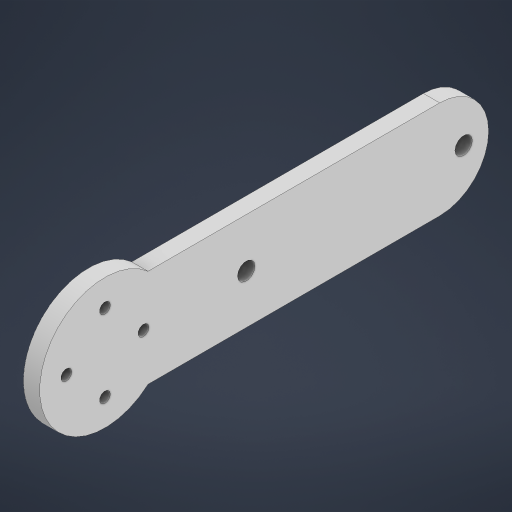
# Autodesk Inventor part: union_servos_2
Saved by Autodesk Inventor 2023.1 (Build 271208000, 208)
## iProperties
Created: 2022-11-07
Part Number: union_servos_2
Material: Generic
Document SubType Name: Modeling
Designer: amtat
Density: 1 g/cm^3
Appearance: Default
Author: amtat
Autodesk Inventor part; units mm, degrees
ref_plane "YZ Plane" through (0, 0, 0) normal (1, 0, 0) x (0, 1, 0)
ref_plane "XZ Plane" through (0, 0, 0) normal (0, 1, 0) x (-1, 0, 0)
ref_plane "XY Plane" through (0, 0, 0) normal (0, 0, 1) x (1, 0, 0)
sketch "Sketch1" plane through (0, 0, 0) normal (1, 0, 0) x (0, 1, 0)
  circle A0 centre (0, 0) radius 1.6
  line L0 (0, 0) -> (0, -40)
  circle A1 centre (0, -40) radius 1.6
  line L1 (0, -40) -> (0, -44.6)
  line L2 (0, -44.6) -> (0, -35.6)
  line L3 (0, 0) -> (0, 4.6)
  line L4 (0, 4.6) -> (0, -4.4)
  circle A2 centre (0, -35.6) radius 9
  line L5 (9, -4.4) -> (9, -35.6)
  line L6 (-9, -35.6) -> (-9, -4.4)
  line L7 (0, 0) -> (0, 7)
  line L8 (0, 7) -> (9, 7)
  line L9 (9, 7) -> (9, -4.4)
  line L10 (0, 7) -> (-9, 7)
  line L11 (-9, 7) -> (-9, -4.4)
  dimension "d0" = 3.2
  dimension "d1" = 40
  dimension "d2" = 3.2
  dimension "d3" = 4.6
  dimension "d4" = 9
  dimension "d5" = 4.6
  dimension "d6" = 9
  dimension "d9" = 7
  constraints: 24 end point, 4 point on line, 3 centre point, 3 coincident, 3 perpendicular, 3 point on circle, 3 vertical, 1 tangent
  measures "d0" diameter of A0
  measures "d1" distance of L0.start L0.end
  measures "d2" diameter of A1
  measures "d3" distance of L1.start L1.end
  measures "d4" distance of L1.end L2.end
  measures "d5" distance of L0.start L3.end
  measures "d6" distance of L3.end L4.end
  measures "d9" distance of L0.start L7.end
extrude "Extrusion2" add sketch "Sketch1" along normal blind 3 contours A0 L3 L7 L8 L9 L5 A2 L0 | A0 L0 A2 L6 L11 L10 L7 L3 | A2 L1 A1 L0 | L0 A1 L1 A2
sketch "Sketch2" plane through (0, -9, 7) normal (0, 0, 1) x (1, 0, 0)
  line L0 (0, 18) -> (0, 0) projected
  line L1 (0, 0) -> (3, 0) projected
  line L2 (3, 18) -> (3, 0) projected
  line L3 (0, 18) -> (3, 18) projected
  point P0 (0, 9)
extrude "Extrusion3" add sketch "Sketch2" along normal blind 24.5
sketch "Sketch5" plane through (3, 0, 0) normal (1, 0, 0) x (0, 0, -1)
  line L0 (35.6, 9) -> (-31.5, 9) projected
  line L1 (-31.5, -9) -> (-31.5, 9) projected
  line L2 (35.6, -9) -> (-31.5, -9) projected
  arc A0 (35.6, -9) -> (35.6, 9) centre (35.6, 0) ccw projected
  circle A1 centre (40, 0) radius 1.6 projected
  circle A2 centre (0, 0) radius 1.6 projected
  line L3 (0, 0) -> (-10, 0)
  line L4 (-10, 0) -> (-10, 9)
  line L5 (35.6, 9) -> (-31.5, 9) projected
  line L6 (-10, 0) -> (-10, -9)
  line L7 (35.6, -9) -> (-31.5, -9) projected
  line L8 (-10, -9) -> (-14, -9)
  line L9 (-14, -9) -> (-14, 9)
  line L10 (-10, 9) -> (-14, 9)
  dimension "d18" = 10
  dimension "d19" = 4
  constraints: 12 end point, 5 point on line, 2 perpendicular, 1 collinear, 1 horizontal
  measures "d18" distance of L3.start L3.end
  measures "d19" distance of L6.end L8.end
extrude "Extrusion5" add sketch "Sketch5" along normal blind 4.3 contours L4 L6 L2 L9 L0
sketch "Sketch6" plane through (7.3, 0, 0) normal (1, 0, 0) x (0, 0, -1)
  line L0 (-14, -9) -> (-10, -9) projected
  line L1 (-10, -9) -> (-10, 9) projected
  line L2 (-10, 9) -> (-14, 9) projected
  line L3 (-14, 9) -> (-14, -9) projected
  line L4 (-14, -9) -> (-14, 9) projected
  line L5 (-14, 9) -> (-14, 0)
  line L6 (-14, 0) -> (-26, 0)
  circle A0 centre (-26, 0) radius 12
  line L7 (-14, 9) -> (-18.0627, 9)
  line L8 (-14, 9) -> (-31.5, 9) projected
  line L9 (-14, -9) -> (-18.0627, -9)
  line L10 (-14, -9) -> (-31.5, -9) projected
  point P0 (0, 0)
  dimension "d22" = 12
  constraints: 8 end point, 3 point on circle, 2 point on line, 1 centre point, 1 coincident, 1 midpoint, 1 perpendicular
  measures "d22" distance of L5.end L6.end
extrude "Extrusion6" add sketch "Sketch6" along normal blind 3
sketch "Sketch7" plane through (0, 0, 0) normal (-1, 0, 0) x (0, 0, 1)
  line L0 (10, -9) -> (10, 9) projected
  line L1 (14, 9) -> (14, -9) projected
  line L2 (-35.6, 9) -> (31.5, 9) projected
  line L3 (-35.6, 9) -> (31.5, 9) projected
  arc A0 (-35.6, 9) -> (-35.6, -9) centre (-35.6, 0) ccw projected
  line L4 (-35.6, -9) -> (31.5, -9) projected
  line L5 (31.5, 9) -> (31.5, -9) projected
  circle A1 centre (-40, 0) radius 1.6 projected
  circle A2 centre (0, 0) radius 1.6 projected
extrude "Extrusion7" add sketch "Sketch7" along normal blind 2.7 contours L0 L2 L1 L4
sketch "Sketch8" plane through (-2.7, 0, 0) normal (-1, 0, 0) x (0, 0, 1)
  line L0 (14, -9) -> (14, 9) projected
  line L1 (14, 9) -> (10, 9) projected
  line L2 (10, 9) -> (10, -9) projected
  line L3 (10, -9) -> (14, -9) projected
  line L4 (14, 9) -> (14, -9) projected
  line L5 (18.0627, -9) -> (14, -9) projected
  arc A0 (18.0627, -9) -> (18.0627, 9) centre (26, 0) ccw projected
  line L6 (14, 9) -> (18.0627, 9) projected
  point P0 (0, 0)
extrude "Extrusion8" add sketch "Sketch8" along normal blind 3
sketch "Sketch9" plane through (0, -9, 31.5) normal (0, 0, 1) x (1, 0, 0)
  line L0 (0, 18) -> (0, 0) projected
  line L1 (0, 0) -> (3, 0) projected
  line L2 (3, 0) -> (3, 18) projected
  line L3 (3, 18) -> (0, 18) projected
  point P0 (0, 9)
extrude "Extrusion9" cut sketch "Sketch9" against normal blind 17.5
sketch "Sketch10" plane through (10.3, 0, 0) normal (1, 0, 0) x (0, 0, -1)
  line L0 (-18.0627, -9) -> (-10, -9) projected
  line L1 (-10, -9) -> (-10, 9) projected
  line L2 (-10, 9) -> (-18.0627, 9) projected
  arc A0 (-18.0627, 9) -> (-18.0627, -9) centre (-26, 0) ccw projected
  circle A1 centre (-26, 0) radius 12
  line L3 (-26, 0) -> (-18.9, 0)
  line L4 (-26, 0) -> (-26, -7.1)
  circle A2 centre (-18.9, 0) radius 1
  circle A3 centre (-26, -7.1) radius 1
  circle A4 centre (-33.1, 0) radius 1
  circle A5 centre (-26, 7.1) radius 1
  point P0 (0, 0)
  dimension "d31" = 7.1
  dimension "d32" = 7.1
  dimension "d33" = 2
  dimension "d34" = 2
  constraints: 5 centre point, 4 end point, 3 coincident, 2 symmetric about line, 1 concentric, 1 horizontal, 1 vertical, 2 other
  measures "d31" distance of L3.start L3.end
  measures "d32" distance of L3.start L4.end
  measures "d33" diameter of A2
  measures "d34" diameter of A3
extrude "Extrusion10" cut sketch "Sketch10" against normal blind 17.5 contours A2 | A3 | A4 | A5
sketch "Sketch11" plane through (-5.7, 0, 0) normal (-1, 0, 0) x (0, 0, 1)
  circle A0 centre (26, -7.1) radius 1 projected
  circle A1 centre (26, 7.1) radius 1 projected
  circle A2 centre (33.1, 0) radius 1 projected
  circle A3 centre (18.9, 0) radius 1 projected
  line L0 (18.0627, 9) -> (10, 9) projected
  line L1 (10, 9) -> (10, -9) projected
  line L2 (10, -9) -> (18.0627, -9) projected
  arc A4 (18.0627, -9) -> (18.0627, 9) centre (26, 0) ccw projected
  point P0 (0, 0)
extrude "Extrusion11" add sketch "Sketch11" along normal blind 1.7
sketch "Sketch12" plane through (-2.7, 0, 0) normal (1, 0, 0) x (0, 0, -1)
  circle A0 centre (-26, -7.1) radius 1 projected
  circle A1 centre (-26, 7.1) radius 1 projected
  circle A2 centre (-33.1, 0) radius 1 projected
  circle A3 centre (-18.9, 0) radius 1 projected
  line L0 (-18.0627, -9) -> (-10, -9) projected
  line L1 (-10, -9) -> (-10, 9) projected
  line L2 (-10, 9) -> (-18.0627, 9) projected
  arc A4 (-18.0627, 9) -> (-18.0627, -9) centre (-26, 0) ccw projected
  circle A5 centre (-26, -7.1) radius 1 projected
  circle A6 centre (-26, 7.1) radius 1 projected
  circle A7 centre (-33.1, 0) radius 1 projected
  circle A8 centre (-18.9, 0) radius 1 projected
  line L3 (-14, -9) -> (-14, 9) projected
  line L4 (-18.0627, 9) -> (-14, 9) projected
  arc A9 (-18.0627, 9) -> (-18.0627, -9) centre (-26, 0) ccw projected
  line L5 (-14, -9) -> (-18.0627, -9) projected
  point P0 (0, 0)
extrude "Extrusion12" cut sketch "Sketch12" against normal blind 1.7 contours A4 L2 L3 L0
sketch "Sketch13" plane through (10.3, 0, 0) normal (1, 0, 0) x (0, 0, -1)
  circle A0 centre (-26, -7.1) radius 1 projected
  circle A1 centre (-26, 7.1) radius 1 projected
  circle A2 centre (-33.1, 0) radius 1 projected
  circle A3 centre (-18.9, 0) radius 1 projected
  line L0 (-18.0627, -9) -> (-10, -9) projected
  line L1 (-10, -9) -> (-10, 9) projected
  line L2 (-10, 9) -> (-18.0627, 9) projected
  arc A4 (-18.0627, 9) -> (-18.0627, -9) centre (-26, 0) ccw projected
  point P0 (0, 0)
extrude "Extrusion13" add sketch "Sketch13" along normal blind 1.7
sketch "Sketch14" plane through (7.3, 0, 0) normal (-1, 0, 0) x (0, 0, 1)
  line L0 (10, -9) -> (10, 9) projected
  line L1 (10, 9) -> (18.0627, 9) projected
  arc A0 (18.0627, -9) -> (18.0627, 9) centre (26, 0) ccw projected
  line L2 (18.0627, -9) -> (10, -9) projected
  circle A1 centre (18.9, 0) radius 1 projected
  circle A2 centre (33.1, 0) radius 1 projected
  circle A3 centre (26, 7.1) radius 1 projected
  circle A4 centre (26, -7.1) radius 1 projected
  circle A5 centre (26, -7.1) radius 1 projected
  circle A6 centre (26, 7.1) radius 1 projected
  circle A7 centre (33.1, 0) radius 1 projected
  circle A8 centre (18.9, 0) radius 1 projected
  line L3 (14, 9) -> (14, -9) projected
  line L4 (18.0627, -9) -> (14, -9) projected
  arc A9 (18.0627, -9) -> (18.0627, 9) centre (26, 0) ccw projected
  line L5 (14, 9) -> (18.0627, 9) projected
  point P0 (0, 0)
extrude "Extrusion14" cut sketch "Sketch14" against normal blind 1.7 contours L3 L1 A0 L2
sketch "Sketch15" plane through (3, 0, 0) normal (1, 0, 0) x (0, 0, -1)
  circle A0 centre (0, 0) radius 1.6 projected
  circle A1 centre (40, 0) radius 1.6 projected
  line L0 (-10, 9) -> (-10, -9) projected
  line L1 (35.6, -9) -> (-10, -9) projected
  arc A2 (35.6, -9) -> (35.6, 9) centre (35.6, 0) ccw projected
  line L2 (35.6, 9) -> (-10, 9) projected
extrude "Extrusion15" add sketch "Sketch15" along normal blind 9
sketch "Sketch16" plane through (0, 0, 0) normal (-1, 0, 0) x (0, 0, 1)
  line L0 (10, -9) -> (10, 9) projected
  line L1 (-35.6, 9) -> (10, 9) projected
  arc A0 (-35.6, 9) -> (-35.6, -9) centre (-35.6, 0) ccw projected
  line L2 (-35.6, -9) -> (10, -9) projected
  circle A1 centre (-40, 0) radius 1.6 projected
  circle A2 centre (0, 0) radius 1.6 projected
extrude "Extrusion16" cut sketch "Sketch16" against normal blind 9
sketch "Sketch17" plane through (-7.4, 0, 0) normal (-1, 0, 0) x (0, 0, 1)
  line L0 (10, 9) -> (10, -9) projected
  line L1 (10, -9) -> (18.0627, -9) projected
  arc A0 (18.0627, -9) -> (18.0627, 9) centre (26, 0) ccw projected
  line L2 (18.0627, 9) -> (10, 9) projected
  circle A1 centre (18.9, 0) radius 1 projected
  circle A2 centre (33.1, 0) radius 1 projected
  circle A3 centre (26, 7.1) radius 1 projected
  circle A4 centre (26, -7.1) radius 1 projected
  point P0 (0, 0)
extrude "Extrusion17" cut sketch "Sketch17" against normal blind 16.4
body "Solid2"
